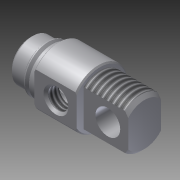
# Autodesk Inventor part: 007P0Y000_rear_head
Saved by Autodesk Inventor 2012 (Build 160160000, 160)
## iProperties
Created: 2013-01-17
Part Number: 007P0Y000_rear_head
Material: Default
Catalog Web Link: www.cadenas.de
Description: Rear Head-Original Line - Standard Air Cylinders
Vendor: BIMBA
Document SubType Name: Modeling
Designer: William
Manufacturer: BIMBA
Density: 1 g/cm^3
Category: PARTsolutions
Company: BIMBA
Title: 007P0Y000_rear_head
Author: Cadenas PARTsolutions
Comments: Original Line - Standard Air Cylinders
PSOL_IDENT_0: {\\10.0.0.242\data_v9\23d-libs\bimba\bimba\bimba_imperial\bimba_full_line\original_line_cylinders\st
PSOL_IDENT_1: andard_air_cylinders\rear_head.prj},233 {VTYP=3D},{NB=007P0Y000_rear_head},{LINA=007P0Y000_rear_head
PSOL_IDENT_2: },{NN=Rear Head},{DATE=24.09.2012 07:58:44},{GEOMDATE=24.09.2012 00:00:00},{VERSION=},{LINEID=10},{L
PSOL_IDENT_3: INESUBID=-1},{WBVAR=MNT,ACTING,DER,Q,T1,T2,T3,T4,TRIM,Y,K,MB,CUSH,FBON}  {NB=007P0Y000_rear_head},{L
PSOL_IDENT_4: INA=007P0Y000_rear_head},{KT=DUMMY},{PN=007P0Y000},{BORE=0.31250},{BOREPN=007},{MNT=P},{MNTALG='' ,
PSOL_IDENT_5: 'Front Nose' , 'P' , 'Rear Pivot'},{ACTING=},{ACTINGALG= '' , 'Single Acting' },{DER=},{DERALG= '' ,
PSOL_IDENT_6: 'Standard' },{Q=},{T1=},{T2=},{T3=},{T4=},{TRIM=0},{Y=Y},{K=},{KALG= '', 'without K', 'K', 'with K'
PSOL_IDENT_7: },{MB=0},{A1=0.8750},{A1N=0.3280},{A1P=0.8750},{A1B=0.0000},{A1S=0.0000},{A2=0.1585},{A2N=0.1585},{
PSOL_IDENT_8: A3=0.0220},{D1=0.4380},{D1N=0.3590},{D1P=0.4380},{D1B=0.0000},{D2=0.3215},{C1=0.0200},{C2=0.0200},{N
PSOL_IDENT_9: DM=0.1900},{TAB=UNF},{NDMDP=0.2000},{D3=0.0000},{A4=0.0000},{A5=0.0000},{D4=0.0000},{A6=0.0000},{A7=
PSOL_IDENT_10: 0.3750},{A8=0.0520},{D5=0.3590},{D6=0.1562},{A9=0.4850},{NDM2=0.3750},{TAB2=UNF},{C11=0.0200},{C22=0
PSOL_IDENT_11: .0100},{C33=0.0100},{C44=0.0100},{A10=0.2500},{A11=0.3975},{NDM3=0.1900},{NDM3N=0.1900},{NDM3B=0.000
PSOL_IDENT_12: 0},{TAB3=UNF},{TAB3N=UNF},{TAB3B=-},{A12=0.375},{A12N=0.3750},{A12B=0.0000},{A13=0.7190},{D7=0.1270}
PSOL_IDENT_13: ,{D8=0.0000},{A14=0.0000},{A15=0.0000},{D9=0.0000},{R1=0.0000},{X1=0.0000},{X2=0.0000},{CX=0.0000},{
PSOL_IDENT_14: CC=0.0000},{CON=1},{S1=0.0000},{DB=0.0000},{X1B=0.0000},{X2B=0.0000},{A8B=0.0000},{A9B=0.0000},{MODE
PSOL_IDENT_15: L=1},{NDM4=0.0000},{TAB4=-},{NDM4DP=0.0000},{BC=0.0000},{B1=0.0000},{B2=0.0000},{B3=0.0000},{ON=0},{
PSOL_IDENT_16: ON2=1},{G1=0.0000},{G2=0.0000},{G3=0.0000},{G4=0.0000},{GD=0.0000},{G5=0.0000},{G6=0.0000},{RON=0},{
PSOL_IDENT_17: H1=0.0000},{H2=0.0000},{H3=0.0000},{H4=0.0000},{H5=0.0000},{H6=0.0000},{F=0.0000},{PNUT=0.5335},{CUS
PSOL_IDENT_18: H=0},{CC11=0.000},{CC111=0.0000},{CC22=0.0000},{CC33=0.0000},{CC44=0.0000},{CC55=0.0000},{CD1=0.0000
PSOL_IDENT_19: },{CD2=0.0000},{CD3=0.0000},{CNDM3=0.0000},{CTAB3=0.0000},{OLEN=0.7190},{OD=0.1895},{STDIS=0.0000},{
PSOL_IDENT_20: STDIS1=0.0000},{BUSHCON=D-25359},{BUSHL=0.2500},{FBON=0},{LCD=0.0000}
CNS_NT: Original Line - Standard Air Cylinders
CNS_NB: 007P0Y000_rear_head
CNS_NBSYN: $PN._rear_head
CNS_LINA: 007P0Y000_rear_head
CNS_PN: 007P0Y000
CNS_BORE: 0.31250
CNS_BOREPN: 007
CNS_MNT: Rear Pivot
CNS_MNTALG: '' , 'Front Nose' , 'P' , 'Rear Pivot'
CNS_ACTING: Single Acting
CNS_ACTINGALG: '' , 'Single Acting'
CNS_DER: Standard
CNS_DERALG: '' , 'Standard'
CNS_Q: Without Side Ported Rear Head
CNS_T1: without T1
CNS_T2: without T2
CNS_T3: without T3
CNS_T4: without T4
CNS_TRIM: 0
CNS_Y: with Pivot Bushing
CNS_K: without K
CNS_KALG: '', 'without K', 'K', 'with K'
CNS_MB: 0
CNS_A1: 0.8750
CNS_A1N: 0.3280
CNS_A1P: 0.8750
CNS_A1B: 0.0000
CNS_A1S: 0.0000
CNS_A2: 0.159
CNS_A2N: 0.1585
CNS_A3: 0.0220
CNS_D1: 0.4380
CNS_D1N: 0.3590
CNS_D1P: 0.4380
CNS_D1B: 0.0000
CNS_D2: 0.3215
CNS_C1: 0.0200
CNS_C2: 0.0200
CNS_NDM: 0.1900
CNS_TAB: UNF
CNS_NDMDP: 0.2000
CNS_D3: 0.0000
CNS_A4: 0.0000
CNS_A5: 0.0000
CNS_D4: 0.0000
CNS_A6: 0.0000
CNS_A7: 0.3750
CNS_A8: 0.0520
CNS_D5: 0.3590
CNS_D6: 0.1562
CNS_A9: 0.4850
CNS_NDM2: 0.3750
CNS_TAB2: UNF
CNS_C11: 0.0200
CNS_C22: 0.0100
CNS_C33: 0.0100
CNS_C44: 0.0100
CNS_A10: 0.2500
CNS_A11: 0.3975
CNS_NDM3: 0.1900
CNS_NDM3N: 0.1900
CNS_NDM3B: 0.0000
CNS_TAB3: UNF
CNS_TAB3N: UNF
CNS_TAB3B: -
CNS_A12: 0.375
CNS_A12N: 0.3750
CNS_A12B: 0.0000
CNS_A13: 0.7190
CNS_D7: 0.1270
CNS_D8: 0.0000
CNS_A14: 0.0000
CNS_A15: 0.0000
CNS_D9: 0.0000
CNS_R1: 0.0000
CNS_X1: 0.0000
CNS_X2: 0.0000
CNS_CX: 0.0000
CNS_CC: 0.0000
CNS_CON: 1
CNS_S1: 0.0000
CNS_DB: 0.0000
CNS_X1B: 0.0000
CNS_X2B: 0.0000
CNS_A8B: 0.0000
CNS_A9B: 0.0000
CNS_MODEL: 1
CNS_NDM4: 0.0000
CNS_TAB4: -
CNS_NDM4DP: 0.0000
CNS_BC: 0.0000
CNS_B1: 0.0000
CNS_B2: 0.0000
CNS_B3: 0.0000
CNS_ON: 0
CNS_ON2: 1
CNS_G1: 0.0000
CNS_G2: 0.0000
CNS_G3: 0.0000
CNS_G4: 0.0000
CNS_GD: 0.0000
CNS_G5: 0.0000
CNS_G6: 0.0000
CNS_RON: 0
CNS_H1: 0.0000
CNS_H2: 0.0000
CNS_H3: 0.0000
CNS_H4: 0.0000
CNS_H5: 0.0000
CNS_H6: 0.0000
CNS_F: 0.0000
CNS_PNUT: 0.5335
CNS_CUSH: 0
CNS_CC11: 0.000
CNS_CC111: 0.0000
CNS_CC22: 0.0000
CNS_CC33: 0.0000
CNS_CC44: 0.0000
CNS_CC55: 0.0000
CNS_CD1: 0.0000
CNS_CD2: 0.0000
CNS_CD3: 0.0000
CNS_CNDM3: 0.0000
CNS_CTAB3: 0.0000
CNS_OLEN: 0.7190
CNS_OD: 0.1895
CNS_STDIS: 0.0000
CNS_STDIS1: 0.0000
CNS_BUSHCON: D-25359
CNS_BUSHL: 0.2500
CNS_FBON: 0
CNS_LCD: 0.0000
SUPPLIER: BIMBA
ARTICLENO: 007P0Y000_rear_head
BOMINFO: 007P0Y000_rear_head
CREATOR: CADENAS GmbH
Autodesk Inventor part; units mm, degrees
sketch "Sketch_8" plane through (0, 0, 0) normal (0, 0, 1) x (1, 0, 0)
  line L0 (13.5509, 0) -> (0, 0)
  line L1 (0, 0) -> (0, 3.5751)
  line L2 (0, 3.5751) -> (0.508, 4.0831)
  line L3 (0.508, 4.0831) -> (2.9083, 4.0831)
  line L4 (2.9083, 4.0831) -> (3.4671, 3.5242)
  line L5 (3.4671, 3.5242) -> (4.0259, 3.5242)
  line L6 (4.0259, 3.5242) -> (4.0259, 4.3053)
  line L7 (4.0259, 4.3053) -> (4.2799, 4.5593)
  line L8 (4.2799, 4.5593) -> (5.3467, 4.5593)
  line L9 (5.3467, 4.5593) -> (5.3467, 5.3086)
  line L10 (5.3467, 5.3086) -> (5.6007, 5.5626)
  line L11 (5.6007, 5.5626) -> (13.2969, 5.5626)
  line L12 (13.2969, 5.5626) -> (13.5509, 5.3086)
  line L13 (13.5509, 5.3086) -> (13.5509, 0)
  line L14 (13.5509, 0) -> (0, 0)
  constraints: 30 end point
revolve "Revolution1" add sketch "Sketch_8" angle 360 about axis through (13.5509, 0, 0) along (1, 0, 0)
sketch "Sketch_14" plane through (0, 0, 0) normal (0, 0, 1) x (1, 0, 0)
  line L0 (22.225, 0) -> (13.5509, 0)
  line L1 (13.5509, 0) -> (13.5509, 4.7625)
  line L2 (13.5509, 4.7625) -> (21.5951, 4.7625)
  line L3 (21.5951, 4.7625) -> (22.225, 4.1326)
  line L4 (22.225, 4.1326) -> (22.225, 0)
  line L5 (22.225, 0) -> (13.5509, 0)
  constraints: 12 end point
revolve "Revolution2" add sketch "Sketch_14" angle 360 about axis through (22.225, 0, 0) along (1, 0, 0)
thread "Thread1" size "3/8-24 UNF" class "2A" standard "ANSI Unified Screw Threads" full length
sketch "Sketch_9" plane through (22.225, 0, 0) normal (1, 0, 0) x (0, 0, -1)
  line L0 (-11.1252, -22.2504) -> (11.1252, -22.2504)
  line L1 (11.1252, -22.2504) -> (11.1252, 22.2504)
  line L2 (11.1252, 22.2504) -> (-11.1252, 22.2504)
  line L3 (-11.1252, 22.2504) -> (-11.1252, -22.2504)
  line L4 (-3.175, -11.1252) -> (3.175, -11.1252)
  line L5 (3.175, -11.1252) -> (3.175, 11.1252)
  line L6 (3.175, 11.1252) -> (-3.175, 11.1252)
  line L7 (-3.175, 11.1252) -> (-3.175, -11.1252)
  constraints: 16 end point
extrude "Extrusion1" cut sketch "Sketch_9" against normal blind 8.6741
sketch "Sketch_44" plane through (13.5509, 0, 0) normal (1, 0, 0) x (0, 0, -1)
  line L0 (-10.0965, 5.5626) -> (-10.0965, -5.5626)
  line L1 (-10.0965, -5.5626) -> (-4.5339, -5.5626)
  line L2 (-4.5339, -5.5626) -> (-4.5339, 5.5626)
  line L3 (-4.5339, 5.5626) -> (-10.0965, 5.5626)
  constraints: 8 end point
extrude "Extrusion2" cut sketch "Sketch_44" against normal blind 8.2042
sketch "Sketch5" plane through (0, 0, 0) normal (-1, 0, 0) x (0, 0, 1)
  point P0 (0, 0)
hole "Drilling 1" at (0, 0, 0) direction (1, 0, 0) diameter 3.9675 depth 12.319 tip angle 120
sketch "Sketch6" plane through (5.6007, 3.2228, 4.5339) normal (0, 0, 1) x (1, 0, 0)
  point P0 (3.9243, -3.2228)
hole "Drilling 2" at (9.525, 0, 4.5339) direction (0, 0, -1) diameter 3.9624 depth 4.5339 countersink diameter 4.826 countersink angle 90 thread size "10-32 UNF" class "2B" standard "ANSI Unified Screw Threads"
sketch "Sketch_24" plane through (0, 0, 0) normal (0, 0, 1) x (1, 0, 0)
  line L0 (4.0259, 0) -> (3.4671, 0)
  line L1 (3.3065, 4.4751) -> (3.9121, 3.8695)
  arc A0 (3.9121, 3.6899) -> (3.9121, 3.8695) centre (3.8223, 3.7797) ccw
  line L2 (3.9121, 3.6899) -> (3.7465, 3.5242)
  line L3 (3.7465, 3.5242) -> (3.4671, 3.5242)
  line L4 (3.4671, 3.5242) -> (3.4671, 3.2702)
  line L5 (3.4671, 3.2702) -> (4.0259, 3.2702)
  line L6 (4.0259, 3.2702) -> (4.0259, 4.0431)
  line L7 (4.0259, 4.0431) -> (3.5097, 4.5593)
  line L8 (3.5097, 4.5593) -> (3.3065, 4.5593)
  line L9 (3.3065, 4.5593) -> (3.3065, 4.4751)
  constraints: 20 end point, 2 point on circle, 1 centre point
revolve "Revolution3" add sketch "Sketch_24" angle 360 about axis through (4.0259, 0, 0) along (1, 0, 0)
sketch "Sketch_43" plane through (0, 0, 0) normal (0, 0, 1) x (1, 0, 0)
  circle A0 centre (18.2626, 0) radius 2.4066
  constraints: 1 centre point
extrude "Extrusion3" cut sketch "Sketch_43" along normal mid plane 9.525
ref_plane "to_tube_XY" through (3.4671, 0, 0) normal (1, 0, 0) x (0, 0, -1)
ref_plane "to_tube_YZ" through (3.4671, 0, 0) normal (0, 0, -1) x (0, 1, 0)
ref_plane "to_tube_ZX" through (3.4671, 0, 0) normal (0, 1, 0) x (1, 0, 0)
ref_plane "to_nut_XY" through (13.5509, 0, 0) normal (1, 0, 0) x (0, 0, -1)
ref_plane "to_nut_YZ" through (13.5509, 0, 0) normal (0, 0, -1) x (0, 1, 0)
ref_plane "to_nut_ZX" through (13.5509, 0, 0) normal (0, 1, 0) x (1, 0, 0)
ref_plane "lovra1_XY" through (22.225, 0, 0) normal (1, 0, 0) x (0, 0, -1)
ref_plane "lovra1_YZ" through (22.225, 0, 0) normal (0, 0, -1) x (0, 1, 0)
ref_plane "lovra1_ZX" through (22.225, 0, 0) normal (0, 1, 0) x (1, 0, 0)
ref_plane "lovra2_XY" through (22.225, 0, 0) normal (1, 0, 0) x (0, 0, -1)
ref_plane "lovra2_YZ" through (22.225, 0, 0) normal (0, 0, -1) x (0, 1, 0)
ref_plane "lovra2_ZX" through (22.225, 0, 0) normal (0, 1, 0) x (1, 0, 0)
ref_plane "lovra3_XY" through (22.225, 0, 0) normal (1, 0, 0) x (0, 0, -1)
ref_plane "lovra3_YZ" through (22.225, 0, 0) normal (0, 0, -1) x (0, 1, 0)
ref_plane "lovra3_ZX" through (22.225, 0, 0) normal (0, 1, 0) x (1, 0, 0)
ref_plane "to_pin_XY" through (18.2626, 0, 0) normal (0, 0, 1) x (1, 0, 0)
ref_plane "to_pin_YZ" through (18.2626, 0, 0) normal (1, 0, 0) x (0, 1, 0)
ref_plane "to_pin_ZX" through (18.2626, 0, 0) normal (0, 1, 0) x (0, 0, 1)
ref_plane "olen_XY" through (18.2626, 0, 0) normal (1, 0, 0) x (0, 0, -1)
ref_plane "olen_YZ" through (18.2626, 0, 0) normal (0, 0, -1) x (0, 1, 0)
ref_plane "olen_ZX" through (18.2626, 0, 0) normal (0, 1, 0) x (1, 0, 0)
ref_plane "thd1_XY" through (22.225, 0, 4.7625) normal (1, 0, 0) x (0, 0, -1)
ref_plane "thd1_YZ" through (22.225, 0, 4.7625) normal (0, 0, -1) x (0, 1, 0)
ref_plane "thd1_ZX" through (22.225, 0, 4.7625) normal (0, 1, 0) x (1, 0, 0)
ref_plane "p1_XY" through (22.225, 0, 3.175) normal (1, 0, 0) x (0, 0, -1)
ref_plane "p1_YZ" through (22.225, 0, 3.175) normal (0, 0, -1) x (0, 1, 0)
ref_plane "p1_ZX" through (22.225, 0, 3.175) normal (0, 1, 0) x (1, 0, 0)
ref_plane "thd2_XY" through (22.225, 0, -4.7625) normal (1, 0, 0) x (0, 0, -1)
ref_plane "thd2_YZ" through (22.225, 0, -4.7625) normal (0, 0, -1) x (0, 1, 0)
ref_plane "thd2_ZX" through (22.225, 0, -4.7625) normal (0, 1, 0) x (1, 0, 0)
ref_plane "p2_XY" through (22.225, 0, -3.175) normal (1, 0, 0) x (0, 0, -1)
ref_plane "p2_YZ" through (22.225, 0, -3.175) normal (0, 0, -1) x (0, 1, 0)
ref_plane "p2_ZX" through (22.225, 0, -3.175) normal (0, 1, 0) x (1, 0, 0)
ref_plane "port2_XY" through (22.225, 0, 0) normal (1, 0, 0) x (0, 0, -1)
ref_plane "port2_YZ" through (22.225, 0, 0) normal (0, 0, -1) x (0, 1, 0)
ref_plane "port2_ZX" through (22.225, 0, 0) normal (0, 1, 0) x (1, 0, 0)
ref_plane "port_XY" through (9.525, 0, 0) normal (0, 0, 1) x (1, 0, 0)
ref_plane "port_YZ" through (9.525, 0, 0) normal (1, 0, 0) x (0, 1, 0)
ref_plane "port_ZX" through (9.525, 0, 0) normal (0, 1, 0) x (0, 0, 1)
ref_plane "1_XY" through (13.5509, 0, 0) normal (1, 0, 0) x (0, 0, -1)
ref_plane "1_YZ" through (13.5509, 0, 0) normal (0, 0, -1) x (0, 1, 0)
ref_plane "1_ZX" through (13.5509, 0, 0) normal (0, 1, 0) x (1, 0, 0)
ref_plane "lovra21_XY" through (0, 0, 5.2705) normal (1, 0, 0) x (0, 0, -1)
ref_plane "lovra21_YZ" through (0, 0, 5.2705) normal (0, 0, -1) x (0, 1, 0)
ref_plane "lovra21_ZX" through (0, 0, 5.2705) normal (0, 1, 0) x (1, 0, 0)
ref_plane "lovra22_XY" through (0, 0, -5.2705) normal (1, 0, 0) x (0, 0, -1)
ref_plane "lovra22_YZ" through (0, 0, -5.2705) normal (0, 0, -1) x (0, 1, 0)
ref_plane "lovra22_ZX" through (0, 0, -5.2705) normal (0, 1, 0) x (1, 0, 0)
ref_plane "to_screw_XY" through (9.525, 0, 0) normal (0, 1, 0) x (1, 0, 0)
ref_plane "to_screw_YZ" through (9.525, 0, 0) normal (1, 0, 0) x (0, 0, -1)
ref_plane "to_screw_ZX" through (9.525, 0, 0) normal (0, 0, -1) x (0, 1, 0)
ref_plane "to_mounting_bracket_XY" through (13.5509, 0, 0) normal (1, 0, 0) x (0, 0, -1)
ref_plane "to_mounting_bracket_YZ" through (13.5509, 0, 0) normal (0, 0, -1) x (0, 1, 0)
ref_plane "to_mounting_bracket_ZX" through (13.5509, 0, 0) normal (0, 1, 0) x (1, 0, 0)
body "Solid1"
